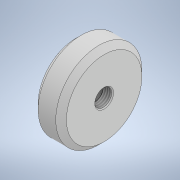
# Autodesk Inventor part: 711132
Saved by Autodesk Inventor 2022 (Build 260153000, 153)
## iProperties
Created: 2021-10-22
Part Number: 711132
Material: Типовые
Document SubType Name: Modeling
Designer: RaNSiD
Density: 1 g/cm^3
Appearance: По умолчанию
Author: RaNSiD
Autodesk Inventor part; units mm, degrees
ref_plane "YZ Plane" through (0, 0, 0) normal (1, 0, 0) x (0, 1, 0)
ref_plane "XZ Plane" through (0, 0, 0) normal (0, 1, 0) x (-1, 0, 0)
ref_plane "XY Plane" through (0, 0, 0) normal (0, 0, 1) x (1, 0, 0)
sketch "Эскиз1" plane through (0, 0, 0) normal (0, 0, 1) x (1, 0, 0)
  line L0 (0, 0) -> (0, 20)
  line L1 (0, 20) -> (2.8284, 22.8284)
  line L2 (0, 20) -> (4, 20) construction
  line L3 (0, 0) -> (15, 0)
  line L4 (15, 0) -> (15, 20)
  line L5 (15, 20) -> (12.1716, 22.8284)
  line L6 (12.1716, 22.8284) -> (2.8284, 22.8284)
  dimension "d0" = 20
  dimension "d1" = 4
  dimension "d2" = 45
  dimension "d3" = 15
  dimension "d4" = 4
  dimension "d5" = 135
  constraints: 14 end point, 2 horizontal, 1 equal length, 1 parallel, 1 perpendicular, 1 vertical
  measures "d0" distance of L0.start L0.end
  measures "d1" distance of L0.end L1.end
  measures "d2" angle of L2 L1
  measures "d3" distance of L0.start L3.end
  measures "d4" distance of L4.end L5.end
  measures "d5" angle of L5 L4
revolve "Вращение1" add sketch "Эскиз1" angle 360 about axis through (0, 0, 0) along (1, 0, 0)
sketch "Эскиз2" plane through (15, 0, 0) normal (1, 0, 0) x (0, 0, -1)
  point P0 (0, 0)
  point P1 (0, 0)
  constraints: 1 coincident
hole "Отверстие1" at (15, 0, 0) direction (-1, 0, 0) diameter 9 depth 5 countersink diameter 10 countersink angle 90
sketch "Эскиз3" plane through (0, 0, 0) normal (0, 0, 1) x (1, 0, 0)
  line L0 (10, -4.5) -> (10, 4.5) projected
  line L1 (10, 5) -> (9.5, 5)
  line L2 (9.5, 5) -> (9.5, 0)
  line L3 (9.5, 0) -> (10, 0)
  line L4 (10, 0) -> (10, 5)
  point P0 (0, 0)
  dimension "d14" = 5
  dimension "d15" = 0.5
  constraints: 8 end point, 2 parallel, 1 horizontal, 1 midpoint, 1 perpendicular
  measures "d14" distance of L1.end L2.end
  measures "d15" distance of L1.start L1.end
revolve "Вращение2" cut sketch "Эскиз3" angle 360 about axis through (9.5, 0, 0) along (1, 0, 0)
sketch "Эскиз4" plane through (0, 0, 0) normal (-1, 0, 0) x (0, 0, 1)
  point P0 (0, 0)
  point P1 (-18, 0)
  point P2 (-9, -15.5885)
  point P3 (9, -15.5885)
  point P4 (18, 0)
  point P5 (9, 15.5885)
  point P6 (-9, 15.5885)
  dimension "d17" = 18
  dimension "d20" = 360
  constraints: 7 other
  measures "d17" distance of point (0, 0) point (-18, 0)
hole "Отверстие2" at (0, 0, -18) at (0, -15.5885, -9) at (0, -15.5885, 9) at (0, 0, 18) at (0, 15.5885, 9) at (0, 15.5885, -9) direction (1, 0, 0) diameter 4 depth 4 tip angle 90
thread "Резьба1" size "M9x1.25" class "6H" standard "ANSI Metric M Profile" full length
